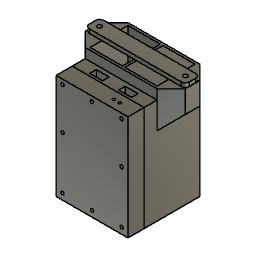
Battery Holder V2 v21 (Autodesk Fusion 360 design; units mm, degrees)
Autodesk Fusion 360 part; units mm, degrees
sketch "Battery" plane through (0, 0, 0) normal (0, 0, 1) x (1, 0, 0)
  line L0 (0, 0) -> (40, 0)
  line L1 (40, 0) -> (40, 47)
  line L2 (40, 47) -> (0, 47)
  line L3 (0, 47) -> (0, 0)
  line L4 (43, 0) -> (83, 0)
  line L5 (83, 0) -> (83, 47)
  line L6 (83, 47) -> (43, 47)
  line L7 (43, 47) -> (43, 0)
  dimension "d1" = 47
  dimension "d2" = 40
  dimension "d5" = 3
  constraint horizontal L0
  constraint vertical L1
  constraint horizontal L2
  constraint vertical L3
  constraint coincident L0.start L3.end
  constraint horizontal L4
  constraint vertical L5
  constraint horizontal L6
  constraint vertical L7
  constraint equal L2 L6
  constraint equal L1 L7
  constraint coincident L0 L4.start
  measures "d1" distance of L0.start L2.end
  measures "d2" distance of L1.end L2.end
  measures "d5" distance of L1 L7
extrude "Battery (1)" add sketch "Battery" along normal blind 138 makes body 1 at (0, 31.3333, 46) makes body 2 at (43, 31.3333, 46)
sketch "Battery Shell" plane through (0, 0, 0) normal (0, 0, -1) x (1, 0, 0)
  line L0 (0, 0) -> (0, -47)
  line L1 (0, -47) -> (40, -47)
  line L2 (40, -47) -> (40, 0)
  line L3 (40, 0) -> (0, 0)
  line L4 (-3, 3) -> (86, 3)
  line L5 (86, 3) -> (86, -50)
  line L6 (86, -50) -> (-3, -50)
  line L7 (-3, -50) -> (-3, 3)
  line L8 (83, 0) -> (83, -47)
  dimension "d8" = 3
  dimension "d9" = 3
  dimension "d10" = 3
  dimension "d12" = 3
  constraint horizontal L4
  constraint vertical L5
  constraint horizontal L6
  constraint vertical L7
  measures "d8" distance of L3 L4
  measures "d9" distance of L1 L6
  measures "d10" distance of L0 L7
  measures "d12" distance of L5 L8
extrude "Bottom Holder" add sketch "Battery Shell" along normal blind 4 separate body contours L0 L1 L2 L3 | L4 L5 L6 L7 makes body 3
extrude "Bat Holder Upper Extrusion" add 1 faces at (26.6667, 32.3333, 0) along direction (0, 0, 1) up to surface (138 mm away) separate body on bodies 3 makes body 4
combine "Combine1" operation add target body 3 tool bodies 4
combine "Combine2" operation cut target body 3 tool bodies 2 1 keep tools
sketch "Bat Holder Left Cell Bottom Air Holes" plane through (0, 0, 0) normal (0, 0, 1) x (-1, 0, 0)
  line L0 (0, -47) -> (0, 0)
  line L1 (0, 0) -> (-40, 0)
  line L2 (-40, 0) -> (-40, -47)
  line L3 (-40, -47) -> (0, -47)
  line L4 (-83, -47) -> (-83, 0) construction
  line L5 (-43, 0) -> (-43, -47) construction
  line L6 (0, -23.5) -> (-40, -23.5) construction
  line L7 (-20, -23.5) -> (-20, -47) construction
  line L8 (-20, -23.5) -> (-20, 0) construction
  circle A0 centre (-20, -35.25) radius 2
  circle A1 centre (-20, -11.75) radius 2
  dimension "d24" = 4
  constraint midpoint L0 L6.start
  constraint midpoint L2 L6.end
  constraint midpoint L6 L7.start
  constraint midpoint L3 L7.end
  constraint midpoint L1 L8.end
  constraint midpoint L7 A0.centre
  constraint midpoint L8 A1.centre
  constraint equal A0 A1
  measures "d24" diameter of A0
sketch "Bat Holder Right Cell Bottom Air Holes" plane through (0, 0, 0) normal (0, 0, 1) x (-1, 0, 0)
  line L0 (-43, -47) -> (-43, 0)
  line L1 (-43, 0) -> (-83, 0)
  line L2 (-83, 0) -> (-83, -47)
  line L3 (-83, -47) -> (-43, -47)
  line L4 (-43, -23.5) -> (-83, -23.5) construction
  line L5 (-63, -23.5) -> (-63, -47) construction
  line L6 (-63, -23.5) -> (-63, 0) construction
  circle A0 centre (-63, -11.75) radius 2
  circle A1 centre (-63, -35.25) radius 2
  circle A2 centre (-20, -35.25) radius 2
  constraint midpoint L0 L4.start
  constraint midpoint L2 L4.end
  constraint midpoint L4 L5.start
  constraint midpoint L3 L5.end
  constraint midpoint L1 L6.end
  constraint midpoint L6 A0.centre
  constraint midpoint L5 A1.centre
  constraint equal A0 A1
  constraint equal A1 A2
extrude "Bat Holder Bottom Air Holes" cut sketch "Bat Holder Right Cell Bottom Air Holes" sketch "Bat Holder Left Cell Bottom Air Holes" against normal through all contours A0 | A1 of sketch 2 contours A0 | A1 bodies 3
ref_plane "WorkPlane1" through (41.5, 23.5, 67) normal (1, 0, 0) x (0, -1, 0)
sketch "M5 Screw Holder" plane through (0, 0, 138) normal (0, 0, 1) x (-1, 0, 0)
  line L0 (0, -47) -> (-40, -47)
  line L1 (-40, -47) -> (-40, 0)
  line L2 (-40, 0) -> (0, 0)
  line L3 (0, 0) -> (0, -47)
  line L4 (-43, -47) -> (-83, -47)
  line L5 (-83, -47) -> (-83, 0)
  line L6 (-83, 0) -> (-43, 0)
  line L7 (-43, 0) -> (-43, -47)
  line L8 (-86, 3) -> (-86, -50)
  line L9 (-86, -50) -> (3, -50)
  line L10 (3, -50) -> (3, 3)
  line L11 (3, 3) -> (-86, 3)
  line L12 (3, -23.5) -> (-86, -23.5) construction
  line L13 (3, -50) -> (20.5, -32.5)
  line L14 (20.5, -32.5) -> (20.5, -14.5)
  line L15 (20.5, -14.5) -> (3, 3)
  line L16 (-41.5, 3) -> (-41.5, -50) construction
  line L17 (3, -23.5) -> (20.5, -23.5) construction
  circle A0 centre (11.75, -23.5) radius 4.225
  circle A1 centre (11.75, -23.5) radius 2.5
  dimension "d19" = 8.45
  dimension "d20" = 5
  dimension "d21" = 17.5
  dimension "d23" = 45
  constraint midpoint L10 L12.start
  constraint midpoint L8 L12.end
  constraint coincident L9.end L10.start
  constraint perpendicular L9 L14
  constraint coincident L10.end L11.start
  constraint midpoint L11 L16.start
  constraint midpoint L9 L16.end
  constraint equal L13 L15
  constraint midpoint L14 L17.end
  constraint midpoint L17 A0.centre
  constraint concentric A0 A1
  measures "d19" diameter of A0
  measures "d20" diameter of A1
  measures "d21" distance of L10 L14
  measures "d23" angle of L10 L15
extrude "M5 Screw Holder (1)" add sketch "M5 Screw Holder" against normal blind 45 separate body contours L10 L13 L14 L15 | A0 makes body 5
extrude "M5 Heated Insert Hole" cut sketch "M5 Screw Holder" against normal blind 12.75 contours A0 bodies 5
chamfer "Chamfer1" distance 0.4 angle 45 1 edges at (-7.8109, 21.9722, 138) on bodies 5
sketch "Ear Chamfer" plane through (0, -3, 0) normal (0, -1, 0) x (1, 0, 0)
  line L0 (-3, 138) -> (-3, -4)
  line L1 (-3, -4) -> (86, -4)
  line L2 (86, -4) -> (86, 138)
  line L3 (86, 138) -> (-3, 138)
  line L4 (-3, 93) -> (-20.5, 93)
  line L5 (-20.5, 138) -> (-20.5, 93)
  line L6 (-3, 93) -> (-20.5, 110.5)
  dimension "d31" = 45
  constraint coincident L4.start L6.start
  constraint coincident L5 L6.end
  measures "d31" angle of L4 L6
extrude "Ear Chamfer (1)" cut sketch "Ear Chamfer" against normal through all contours L4 L5 L6 bodies 5
mirror "Mirror1" about plane through (41.5, 23.5, 67) normal (1, 0, 0) of bodies 5 makes body 6
combine "Combine3" operation add target body 3 tool bodies 6 5
sketch "Tie Down" plane through (0, 0, 138) normal (0, 0, 1) x (-1, 0, 0)
  circle A0 centre (11.75, -23.5) radius 4.625
  circle A1 centre (-94.75, -23.5) radius 4.625
  line L0 (0, -47) -> (-40, -47)
  line L1 (-40, -47) -> (-40, 0)
  line L2 (-40, 0) -> (0, 0)
  line L3 (0, 0) -> (0, -47)
  line L4 (-43, -47) -> (-83, -47)
  line L5 (-83, -47) -> (-83, 0)
  line L6 (-83, 0) -> (-43, 0)
  line L7 (-43, 0) -> (-43, -47)
  line L8 (-86, -50) -> (3, -50)
  line L9 (3, -50) -> (20.5, -32.5)
  line L10 (20.5, -32.5) -> (20.5, -14.5)
  line L11 (20.5, -14.5) -> (3, 3)
  line L12 (3, 3) -> (-86, 3)
  line L13 (-86, 3) -> (-103.5, -14.5)
  line L14 (-103.5, -14.5) -> (-103.5, -32.5)
  line L15 (-103.5, -32.5) -> (-86, -50)
  line L16 (-103.5, -14.5) -> (20.5, -14.5)
  line L17 (20.5, -14.5) -> (20.5, -32.5)
  line L18 (20.5, -32.5) -> (-103.5, -32.5)
  line L19 (-103.5, -32.5) -> (-103.5, -14.5)
  circle A2 centre (-94.75, -23.5) radius 2.65
  circle A3 centre (11.75, -23.5) radius 2.65
  dimension "d35" = 5.3
  constraint horizontal L16
  constraint vertical L17
  constraint horizontal L18
  constraint vertical L19
  constraint coincident L9.end L10.start
  constraint coincident L13.end L14.start
  constraint concentric A1 A2
  constraint concentric A0 A3
  constraint equal A2 A3
  measures "d35" diameter of A2
extrude "Tie Down" add sketch "Tie Down" along normal blind 5 separate body contours A0 | A1 | L1 L3 L16 L18 | L3 L10 L16 L17 L18 | L1 L7 L16 L18 | L5 L7 L16 L18 | L5 L14 L16 L18 L19 makes body 7
fillet "Tie Down (1)" radius 5 4 edges at (103.5, 14.5, 140.5) (103.5, 32.5, 140.5) (-20.5, 14.5, 140.5) (-20.5, 32.5, 140.5) on bodies 7
ref_plane "WorkPlane2" through (41.5, 23.5, 118) normal (0, 0, 1) x (1, 0, 0)
sketch "XT60" plane through (0, 0, 118) normal (0, 0, 1) x (1, 0, 0)
  line L0 (86, -3) -> (-3, -3) construction
  line L1 (41.5, -3) -> (41.5, -16.1) construction
  line L2 (31.5, -16.1) -> (15.7, -16.1)
  line L3 (15.7, -16.1) -> (15.7, -8)
  line L4 (15.7, -8) -> (31.5, -8)
  line L5 (31.5, -8) -> (31.5, -16.1)
  line L6 (51.5, -16.1) -> (67.3, -16.1)
  line L7 (67.3, -16.1) -> (67.3, -8)
  line L8 (67.3, -8) -> (51.5, -8)
  line L9 (51.5, -8) -> (51.5, -16.1)
  line L10 (31.5, -16.1) -> (41.5, -16.1) construction
  line L11 (41.5, -16.1) -> (51.5, -16.1) construction
  line L12 (31.5, -8) -> (31.5, -3) construction
  dimension "d42" = 8.1
  dimension "d43" = 15.8
  dimension "d44" = 10
  dimension "d45" = 5
  constraint midpoint L0 L1.start
  constraint perpendicular L0 L1
  constraint horizontal L2
  constraint vertical L3
  constraint horizontal L4
  constraint vertical L5
  constraint horizontal L6
  constraint vertical L7
  constraint horizontal L8
  constraint vertical L9
  constraint perpendicular L1 L10
  constraint perpendicular L9 L11
  constraint equal L10 L11
  constraint equal L4 L8
  constraint equal L5 L9
  constraint coincident L0 L12.end
  constraint perpendicular L0 L12
  measures "d42" distance of L6.end L7.end
  measures "d43" distance of L7.end L8.end
  measures "d44" distance of L1.end L6.start
  measures "d45" distance of L4.end L12.end
extrude "XT 60" add sketch "XT60" along normal blind 8 separate body makes body 8 at (62.0333, -10.7, 118) makes body 9 at (26.2333, -13.4, 118)
sketch "Sketch9" plane through (0, 0, 118) normal (0, 0, -1) x (1, 0, 0)
  line L0 (51.5, 16.1) -> (51.5, 8)
  line L1 (51.5, 8) -> (67.3, 8)
  line L2 (67.3, 8) -> (67.3, 16.1)
  line L3 (67.3, 16.1) -> (51.5, 16.1)
  line L4 (86, 3) -> (-3, 3) construction
  line L5 (70.3, 19.1) -> (12.7, 19.1)
  line L6 (12.7, 19.1) -> (12.7, 3)
  line L7 (12.7, 3) -> (70.3, 3)
  line L8 (70.3, 3) -> (70.3, 19.1)
  line L9 (15.7, 16.1) -> (15.7, 8)
  point P0 (15.7, 16.1)
  dimension "d48" = 3
  dimension "d49" = 3
  dimension "d50" = 3
  constraint horizontal L5
  constraint vertical L6
  constraint horizontal L7
  constraint vertical L8
  constraint coincident L4 L6.end
  measures "d48" distance of P0 L5
  measures "d49" distance of L6 L9
  measures "d50" distance of L2 L8
extrude "Extrude10" add sketch "Sketch9" against normal up to surface (8 mm away) separate body contours L0 L1 L2 L3 | L5 L6 L7 L8 makes body 10
combine "Combine4" operation cut target body 10 tool bodies 9 8
combine "Combine5" operation add target body 3 tool bodies 10
sketch "Recess" plane through (0, 0, 118) normal (0, 0, -1) x (1, 0, 0)
  line L0 (67.3, 8) -> (51.5, 8)
  line L1 (51.5, 8) -> (51.5, 16.1)
  line L2 (51.5, 16.1) -> (67.3, 16.1)
  line L3 (67.3, 16.1) -> (67.3, 8)
  line L4 (31.5, 16.1) -> (31.5, 8)
  line L5 (31.5, 8) -> (15.7, 8)
  line L6 (15.7, 8) -> (15.7, 16.1)
  line L7 (15.7, 16.1) -> (31.5, 16.1)
  line L8 (70.3, 3) -> (70.3, 19.1)
  line L9 (70.3, 19.1) -> (12.7, 19.1)
  line L10 (12.7, 19.1) -> (12.7, 3)
  line L11 (12.7, 3) -> (70.3, 3)
  line L12 (23.6, 16.1) -> (23.6, 8) construction
  line L13 (59.4, 16.1) -> (59.4, 8) construction
  line L14 (30.1, 15.05) -> (17.1, 15.05)
  line L15 (17.1, 15.05) -> (17.1, 9.05)
  line L16 (17.1, 9.05) -> (30.1, 9.05)
  line L17 (30.1, 9.05) -> (30.1, 15.05)
  line L18 (30.1, 15.05) -> (17.1, 9.05) construction
  line L19 (17.1, 15.05) -> (30.1, 9.05) construction
  line L20 (65.9, 15.05) -> (52.9, 15.05)
  line L21 (52.9, 15.05) -> (52.9, 9.05)
  line L22 (52.9, 9.05) -> (65.9, 9.05)
  line L23 (65.9, 9.05) -> (65.9, 15.05)
  line L24 (65.9, 15.05) -> (52.9, 9.05) construction
  line L25 (52.9, 15.05) -> (65.9, 9.05) construction
  point P0 (23.6, 12.05)
  point P1 (59.4, 12.05)
  point P2 (23.6, 12.05)
  point P3 (59.4, 12.05)
  dimension "d53" = 6
  dimension "d54" = 13
  constraint midpoint L7 L12.start
  constraint midpoint L5 L12.end
  constraint midpoint L2 L13.start
  constraint midpoint L0 L13.end
  constraint midpoint L12 P2
  constraint midpoint L13 P3
  constraint horizontal L14
  constraint perpendicular L14 L15
  constraint parallel L14 L16
  constraint parallel L15 L17
  constraint coincident L18 P2
  constraint coincident L19 P2
  constraint coincident P2 P0
  constraint horizontal L20
  constraint perpendicular L20 L21
  constraint parallel L20 L22
  constraint parallel L21 L23
  constraint coincident L24 P3
  constraint coincident L25 P3
  constraint coincident P3 P1
  constraint equal L14 L20
  constraint equal L17 L21
  measures "d53" distance of L14.start L16.end
  measures "d54" distance of L14.start L14.end
extrude "Recess (1)" add sketch "Recess" along normal blind 20 contours L0 L1 L2 L3 | L4 L5 L6 L7 | L8 L9 L10 L11 bodies 3
chamfer "Chamfer2" distance 16.1 angle 45 1 edges at (41.5, -19.1, 98) on bodies 3
sketch "Base Hole" plane through (0, -3, 0) normal (0, -1, 0) x (1, 0, 0)
  line L0 (-3, 138) -> (-3, 93)
  line L1 (-3, 93) -> (-3, -4)
  line L2 (-3, -4) -> (86, -4)
  line L3 (86, -4) -> (86, 93)
  line L4 (86, 93) -> (86, 138)
  line L5 (86, 138) -> (-3, 138)
  line L6 (70.3, 126) -> (70.3, 98)
  line L7 (70.3, 98) -> (12.7, 98)
  line L8 (12.7, 98) -> (12.7, 126)
  line L9 (12.7, 126) -> (70.3, 126)
  line L10 (41.5, -4) -> (41.5, 46) construction
  line L11 (68, 27) -> (15, 27) construction
  line L12 (15, 27) -> (15, 65) construction
  line L13 (15, 65) -> (68, 65) construction
  line L14 (68, 65) -> (68, 27) construction
  line L15 (68, 27) -> (15, 65) construction
  line L16 (15, 27) -> (68, 65) construction
  circle A0 centre (65, 30) radius 3
  circle A1 centre (65, 62) radius 3
  circle A2 centre (18, 62) radius 3
  circle A3 centre (18, 30) radius 3
  point P0 (41.5, 46)
  dimension "d58" = 38
  dimension "d59" = 53
  dimension "d60" = 50
  dimension "d61" = 6
  constraint midpoint L2 L10.start
  constraint perpendicular L2 L10
  constraint horizontal L11
  constraint perpendicular L11 L12
  constraint parallel L11 L13
  constraint parallel L12 L14
  constraint coincident L15 P0
  constraint coincident L16 P0
  constraint coincident P0 L10.end
  constraint equal A2 A3
  constraint equal A1 A3
  constraint equal A0 A3
  constraint tangent L12 A3
  constraint tangent L11 A3
  constraint tangent L12 A2
  constraint tangent L13 A2
  constraint tangent L13 A1
  constraint tangent L14 A1
  constraint tangent L14 A0
  constraint tangent L11 A0
  measures "d58" distance of L11.end L12.end
  measures "d59" distance of L11.start L11.end
  measures "d60" distance of L10.start P0
  measures "d61" diameter of A3
extrude "Extrude12" add sketch "Base Hole" along normal blind 5 contours A0 | A1 | A2 | A3 bodies 3
chamfer "Chamfer3" distance 5 angle 45 4 edges at (62.203, -3, 63.0848) (62.203, -3, 31.0848) (15.203, -3, 31.0848) (15.203, -3, 63.0848) on bodies 3
sketch "Screw Hole Clearance" plane through (0, -8, 0) normal (0, -1, 0) x (1, 0, 0)
  circle A0 centre (65, 62) radius 3
  circle A1 centre (65, 62) radius 1.55
  circle A2 centre (65, 30) radius 1.55
  circle A3 centre (18, 30) radius 1.55
  circle A4 centre (18, 62) radius 1.55
  circle A5 centre (18, 62) radius 3
  circle A6 centre (18, 30) radius 3
  circle A7 centre (65, 30) radius 3
  dimension "d67" = 3.1
  constraint concentric A0 A1
  constraint equal A1 A4
  constraint equal A1 A3
  constraint equal A1 A2
  constraint concentric A4 A5
  constraint concentric A3 A6
  constraint concentric A2 A7
  measures "d67" diameter of A1
extrude "Extrude13" cut sketch "Screw Hole Clearance" against normal up to surface (8 mm away) contours A1 | A2 | A3 | A4 bodies 3
sketch "M3 Heated Insert" plane through (0, -8, 0) normal (0, -1, 0) x (1, 0, 0)
  circle A0 centre (65, 62) radius 1.55
  circle A1 centre (65, 62) radius 3
  circle A2 centre (65, 62) radius 2.6
  circle A3 centre (65, 30) radius 2.6
  circle A4 centre (18, 30) radius 2.6
  circle A5 centre (18, 62) radius 2.6
  circle A6 centre (18, 62) radius 3
  circle A7 centre (18, 30) radius 3
  circle A8 centre (65, 30) radius 3
  dimension "d70" = 5.2
  constraint concentric A0 A2
  constraint equal A2 A3
  constraint equal A2 A5
  constraint equal A2 A4
  constraint concentric A5 A6
  constraint concentric A4 A7
  constraint concentric A3 A8
  measures "d70" diameter of A2
extrude "Extrude14" cut sketch "M3 Heated Insert" against normal blind 3.8 contours A2 | A3 | A4 | A5 bodies 3
sketch "Sketch19" plane through (0, -3, 0) normal (0, -1, 0) x (1, 0, 0)
  circle A0 centre (18, 30) radius 8
  circle A1 centre (65, 62) radius 8
  line L0 (-3, 138) -> (-3, 93)
  line L1 (-3, 93) -> (-3, -4)
  line L2 (-3, -4) -> (86, -4)
  line L3 (86, -4) -> (86, 93)
  line L4 (86, 93) -> (86, 138)
  line L5 (86, 138) -> (-3, 138)
  line L6 (70.3, 126) -> (70.3, 98)
  line L7 (70.3, 98) -> (12.7, 98)
  line L8 (12.7, 98) -> (12.7, 126)
  line L9 (12.7, 126) -> (70.3, 126)
  circle A2 centre (65, 30) radius 8
  circle A3 centre (18, 62) radius 8
  line L10 (12.7, 126) -> (70.3, 126)
  line L11 (12.7, 126) -> (-3, 126)
  line L12 (-3, 126) -> (-3, -4)
  line L13 (-3, -4) -> (12.7, -4)
  line L14 (12.7, -4) -> (12.7, 126)
  line L15 (70.3, 126) -> (86, 126)
  line L16 (86, 126) -> (86, -4)
  line L17 (86, -4) -> (70.3, -4)
  line L18 (70.3, -4) -> (70.3, 126)
  line L19 (12.7, -4) -> (70.3, -4)
  line L20 (70.3, -4) -> (70.3, 11)
  line L21 (70.3, 11) -> (12.7, 11)
  line L22 (12.7, 11) -> (12.7, -4)
  dimension "d115" = 15
  constraint horizontal L11
  constraint vertical L12
  constraint horizontal L13
  constraint vertical L14
  constraint coincident L1.end L2.start
  constraint coincident L8.end L9.start
  constraint horizontal L15
  constraint vertical L16
  constraint horizontal L17
  constraint vertical L18
  constraint coincident L2.end L3.start
  constraint coincident L6.start L9.end
  constraint horizontal L19
  constraint vertical L20
  constraint horizontal L21
  constraint vertical L22
  constraint coincident L18 L20.end
  measures "d115" distance of L17.end L20.end
extrude "Extrude20" add sketch "Sketch19" along normal up to surface (16.1 mm away) contours A0 L14 | A0 L0 L1 L2 L8 A3 L11 L12 L13 L14 L22 | A3 L14 | L2 L14 L18 L19 L20 L21 L22 | A1 L2 L3 L4 L6 A2 L15 L16 L17 L18 L20 | A2 L18 | A1 L18 picked at (11.8, 30) picked at (12.2136, 63.4265) picked at (71.0945, 30.7426) picked at (71.3579, 60.9891) bodies 3
sketch "Sketch20" plane through (0, -19.1, 0) normal (0, -1, 0) x (1, 0, 0)
  line L0 (12.7, 114.1) -> (70.3, 114.1)
  line L1 (70.3, 114.1) -> (70.3, 11)
  line L2 (70.3, 11) -> (12.7, 11)
  line L3 (12.7, 11) -> (12.7, 114.1)
  line L4 (86, 126) -> (-3, 126)
  line L5 (-3, 126) -> (-3, -4)
  line L6 (-3, -4) -> (86, -4)
  line L7 (86, -4) -> (86, 126)
  line L8 (12.7, 11) -> (-3, 11) construction
  line L9 (70.3, 11) -> (86, 11) construction
  line L10 (4.85, 11) -> (4.85, 126) construction
  line L11 (78.15, 11) -> (78.15, 126) construction
  line L12 (78.15, 11) -> (78.15, -4) construction
  line L13 (4.85, 11) -> (4.85, -4) construction
  line L14 (4.85, 3.5) -> (78.15, 3.5) construction
  circle A0 centre (4.85, 3.5) radius 3
  circle A1 centre (78.15, 3.5) radius 3
  circle A2 centre (41.5, 3.5) radius 3
  line L15 (41.5, 114.1) -> (41.5, 126) construction
  line L16 (41.5, 120.05) -> (86, 120.05) construction
  line L17 (41.5, 120.05) -> (-3, 120.05) construction
  circle A3 centre (4.85, 120.05) radius 3
  circle A4 centre (41.5, 120.05) radius 3
  circle A5 centre (78.15, 120.05) radius 3
  circle A6 centre (4.85, 68.5) radius 3
  circle A7 centre (78.15, 68.5) radius 3
  circle A8 centre (41.5, 120.05) radius 2
  circle A9 centre (78.15, 120.05) radius 2
  circle A10 centre (4.85, 120.05) radius 2
  circle A11 centre (4.85, 68.5) radius 2
  circle A12 centre (4.85, 3.5) radius 2
  circle A13 centre (41.5, 3.5) radius 2
  circle A14 centre (78.15, 3.5) radius 2
  circle A15 centre (78.15, 68.5) radius 2
  dimension "d119" = 6
  dimension "d120" = 6
  dimension "d121" = 6
  dimension "d123" = 6
  dimension "d124" = 6
  dimension "d125" = 6
  dimension "d127" = 6
  dimension "d129" = 6
  dimension "d136" = 4
  dimension "d138" = 4
  dimension "d139" = 4
  dimension "d140" = 4
  dimension "d142" = 4
  dimension "d144" = 4
  dimension "d145" = 4
  dimension "d146" = 4
  constraint coincident L2.end L3.start
  constraint coincident L5 L8.end
  constraint perpendicular L5 L8
  constraint coincident L1.end L2.start
  constraint coincident L7 L9.end
  constraint perpendicular L7 L9
  constraint midpoint L8 L10.start
  constraint coincident L4 L10.end
  constraint perpendicular L4 L10
  constraint midpoint L9 L11.start
  constraint coincident L4 L11.end
  constraint perpendicular L4 L11
  constraint coincident L6 L12.end
  constraint perpendicular L6 L12
  constraint coincident L6 L13.end
  constraint perpendicular L6 L13
  constraint midpoint L13 L14.start
  constraint midpoint L12 L14.end
  constraint coincident L14.start A0.centre
  constraint coincident L14.end A1.centre
  constraint midpoint L14 A2.centre
  constraint midpoint L0 L15.start
  constraint midpoint L4 L15.end
  constraint midpoint L15 L16.start
  constraint coincident L7 L16.end
  constraint perpendicular L7 L16
  constraint coincident L5 L17.end
  constraint perpendicular L5 L17
  constraint coincident L10 A3.centre
  constraint coincident L17 A3.centre
  constraint coincident L16.start L17.start
  constraint coincident L16 A5.centre
  constraint coincident L11 A5.centre
  constraint midpoint L10 A6.centre
  constraint midpoint L11 A7.centre
  constraint concentric A5 A9
  constraint concentric A3 A10
  constraint concentric A6 A11
  constraint concentric A0 A12
  constraint concentric A2 A13
  constraint concentric A1 A14
  constraint concentric A7 A15
  measures "d119" diameter of A0
  measures "d120" diameter of A2
  measures "d121" diameter of A1
  measures "d123" diameter of A7
  measures "d124" diameter of A5
  measures "d125" diameter of A4
  measures "d127" diameter of A3
  measures "d129" diameter of A6
  measures "d136" diameter of A15
  measures "d138" diameter of A9
  measures "d139" diameter of A8
  measures "d140" diameter of A10
  measures "d142" diameter of A11
  measures "d144" diameter of A12
  measures "d145" diameter of A13
  measures "d146" diameter of A14
extrude "Extrude21" cut sketch "Sketch20" against normal up to surface (16.1 mm away) contours A8 | A9 | A10 | A11 | A12 | A13 | A14 | A15 bodies 3
extrude "Extrude22" cut sketch "Sketch20" against normal blind 4.8 contours A0 | A1 | A2 | A3 | A4 | A5 | A6 | A7 bodies 3
extrude "Extrude23" add sketch "Sketch20" along normal blind 20 separate body contours L4 L5 L6 L7 | A0 | A1 | A2 | A3 | A4 | A5 | A6 | A7 makes body 11
sketch "Sketch21" plane through (0, -39.1, 0) normal (0, -1, 0) x (1, 0, 0)
  circle A0 centre (78.15, 120.05) radius 2
  circle A1 centre (4.85, 120.05) radius 2
  line L0 (70.3, 11) -> (12.7, 11)
  line L1 (12.7, 11) -> (12.7, 114.1)
  line L2 (12.7, 114.1) -> (70.3, 114.1)
  line L3 (70.3, 114.1) -> (70.3, 11)
  circle A2 centre (4.85, 68.5) radius 2
  circle A3 centre (78.15, 68.5) radius 2
  circle A4 centre (78.15, 3.5) radius 2
  circle A5 centre (41.5, 3.5) radius 2
  circle A6 centre (41.5, 120.05) radius 2
  circle A7 centre (4.85, 3.5) radius 2
  line L4 (86, -4) -> (86, 126)
  line L5 (86, 126) -> (-3, 126)
  line L6 (-3, 126) -> (-3, -4)
  line L7 (-3, -4) -> (86, -4)
  line L8 (12.7, 11) -> (70.3, 11)
  line L9 (70.3, 11) -> (70.3, 114.1)
  line L10 (70.3, 114.1) -> (12.7, 114.1)
  line L11 (12.7, 114.1) -> (12.7, 11)
  constraint horizontal L8
  constraint vertical L9
  constraint horizontal L10
  constraint vertical L11
  constraint coincident L2.end L3.start
  constraint coincident L0.end L1.start
extrude "Extrude24" add sketch "Sketch21" against normal blind 5 contours L0 L1 L2 L3 L8 L9 L10 L11 bodies 11
sketch "Sketch22" plane through (0, 0, 126) normal (0, 0, 1) x (-1, 0, 0)
  line L0 (-86, 19.1) -> (3, 19.1)
  line L1 (3, 19.1) -> (3, 39.1)
  line L2 (3, 39.1) -> (-86, 39.1)
  line L3 (-86, 39.1) -> (-86, 19.1)
  line L4 (-86, 29.1) -> (3, 29.1) construction
  circle A0 centre (-58.5, 29.1) radius 1.65
  circle A1 centre (-66, 29.1) radius 1.65
  dimension "d156" = 3.3
  dimension "d157" = 7.5
  dimension "d158" = 20
  constraint midpoint L3 L4.start
  constraint midpoint L1 L4.end
  constraint coincident L4 A0.centre
  constraint coincident L4 A1.centre
  constraint equal A0 A1
  measures "d156" diameter of A1
  measures "d157" distance of A0.centre A1.centre
  measures "d158" horizontal distance of L2.end A1.centre
extrude "Extrude25" cut sketch "Sketch22" against normal up to surface (11.9 mm away) contours A0 | A1 bodies 11
hidden bodies 1
equation "Wall_Thickness = 3 mm"
equation "d5 = Wall_Thickness"
equation "d8 = Wall_Thickness"
equation "d9 = Wall_Thickness"
equation "d10 = Wall_Thickness"
equation "d12 = Wall_Thickness"
equation "M5_HI_D = 8.45 mm"
equation "M5_HI_L_Tall = 12.75 mm"
equation "d19 = M5_HI_D"
equation "d28 = -M5_HI_L_Tall"
equation "d46 = 15.5 mm - 7.5 mm"
equation "M3_HI_D = 5.2 mm"
equation "M3_HI_L_Tall = 3.8 mm"
equation "d70 = M3_HI_D"
equation "d71 = -M3_HI_L_Tall"
equation "M4_HI_D = 6 mm"
equation "M4_HI_L_Tall = 4.8 mm"
equation "M4_Hole = 4 mm"
equation "d119 = M4_HI_D"
equation "d120 = M4_HI_D"
equation "d121 = M4_HI_D"
equation "d123 = M4_HI_D"
equation "d124 = M4_HI_D"
equation "d125 = M4_HI_D"
equation "d127 = M4_HI_D"
equation "d129 = M4_HI_D"
equation "d136 = M4_Hole"
equation "d138 = M4_Hole"
equation "d139 = M4_Hole"
equation "d140 = M4_Hole"
equation "d142 = M4_Hole"
equation "d144 = M4_Hole"
equation "d145 = M4_Hole"
equation "d146 = M4_Hole"
equation "d150 = -M4_HI_L_Tall"
named bodies: "Battery 1", "Battery 2", "Battery Holder", "Battery Tie Down", "XT 60 Right", "XT 60 Left"
